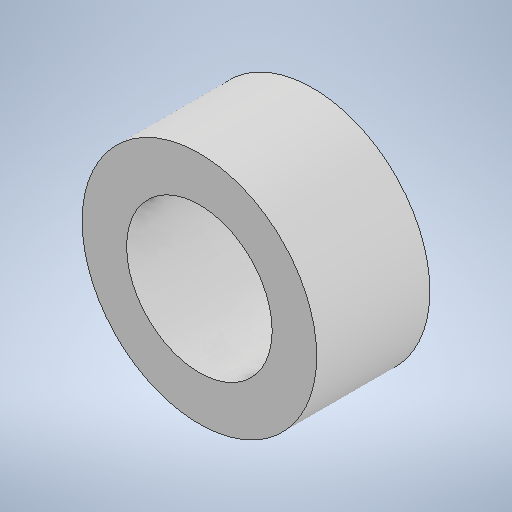
# Autodesk Inventor part: 1103
Saved by Autodesk Inventor 2025.1 (Build 291241000, 241)
## iProperties
Created: 2024-06-07
Part Number: 1103
Material: Generisch
Document SubType Name: Modeling
Designer: ffogue
Density: 1 g/cm^3
Appearance: Vorgabe
Author: ffogue
Autodesk Inventor part; units mm, degrees
ref_plane "YZ Plane" through (0, 0, 0) normal (1, 0, 0) x (0, 1, 0)
ref_plane "XZ Plane" through (0, 0, 0) normal (0, 1, 0) x (-1, 0, 0)
ref_plane "XY Plane" through (0, 0, 0) normal (0, 0, 1) x (1, 0, 0)
sketch "Skizze1" plane through (0, 0, 0) normal (0, 1, 0) x (-1, 0, 0)
  circle A0 centre (0, 0) radius 7.25
  circle A1 centre (0, 0) radius 4.5
  dimension "d0" = 14.5
  dimension "d1" = 9
  constraints: 2 centre point, 2 coincident
  measures "d0" diameter of A0
  measures "d1" diameter of A1
extrude "Extrusion1" add sketch "Skizze1" along normal blind 7
